Autodesk Fusion 360 part; units mm, degrees
note: some values were not read from the file. Set by a fixed rule: which sketch regions a step uses.
(part 12 of 14)
  spline S66 degree 5 poles (-8.0092, 17.6297) (-8.0092, 17.6297) (-8.0093, 17.6299) (-8.0094, 17.6301) (-8.0095, 17.6305) (-8.0098, 17.631) (-8.0101, 17.6317) (-8.0104, 17.6324) (-8.0108, 17.6332) (-8.0112, 17.634) (-8.0117, 17.635) (-8.0122, 17.636) (-8.0127, 17.6371) (-8.0133, 17.6383) (-8.0139, 17.6395) (-8.0146, 17.6408) (-8.0153, 17.6422) (-8.016, 17.6437) (-8.0168, 17.6452) (-8.0176, 17.6469) (-8.0185, 17.6485) (-8.0194, 17.6503) (-8.0203, 17.6521) (-8.0213, 17.654) (-8.0223, 17.6559) (-8.0234, 17.6579) (-8.0245, 17.66) (-8.0256, 17.6621) (-8.0268, 17.6643) (-8.028, 17.6666) (-8.0292, 17.6689) (-8.0305, 17.6713) (-8.0318, 17.6737) (-8.0332, 17.6762) (-8.0346, 17.6788) (-8.0361, 17.6814) (-8.0375, 17.6841) (-8.0391, 17.6868) (-8.0406, 17.6896) (-8.0422, 17.6925) (-8.0438, 17.6954) (-8.0455, 17.6983) (-8.0472, 17.7013) (-8.049, 17.7044) (-8.0508, 17.7075) (-8.0526, 17.7107) (-8.0545, 17.7139) (-8.0564, 17.7172) (-8.0583, 17.7205) (-8.0603, 17.7239) (-8.0623, 17.7273) (-8.0644, 17.7308) (-8.0665, 17.7343) (-8.0686, 17.7378) (-8.0708, 17.7415) (-8.073, 17.7451) (-8.0752, 17.7488) (-8.0775, 17.7526) (-8.0798, 17.7564) (-8.0822, 17.7602) (-8.0846, 17.7641) (-8.087, 17.7681) (-8.0895, 17.772) (-8.092, 17.7761) (-8.0945, 17.7801) (-8.0971, 17.7842) (-8.0997, 17.7884) (-8.1024, 17.7926) (-8.1051, 17.7968) (-8.1078, 17.8011) (-8.1106, 17.8054) (-8.1134, 17.8097) (-8.1162, 17.8141) (-8.1191, 17.8186) (-8.122, 17.823) (-8.125, 17.8276) (-8.128, 17.8321) (-8.131, 17.8367) (-8.1341, 17.8413) (-8.1372, 17.846) (-8.1403, 17.8507) (-8.1435, 17.8554) (-8.1467, 17.8602) (-8.1499, 17.865) (-8.1532, 17.8698) (-8.1565, 17.8747) (-8.1599, 17.8796) (-8.1633, 17.8846) (-8.1667, 17.8896) (-8.1702, 17.8946) (-8.1737, 17.8996) (-8.1772, 17.9047) (-8.1808, 17.9098) (-8.1844, 17.915) (-8.1881, 17.9202) (-8.1918, 17.9254) (-8.1955, 17.9306) (-8.1993, 17.9359) (-8.2031, 17.9412) (-8.2069, 17.9466) (-8.2108, 17.9519) (-8.2147, 17.9573) (-8.2186, 17.9628) (-8.2226, 17.9682) (-8.2266, 17.9737) (-8.2306, 17.9793) (-8.2347, 17.9848) (-8.2388, 17.9904) (-8.243, 17.996) (-8.2472, 18.0016) (-8.2514, 18.0073) (-8.2557, 18.013) (-8.26, 18.0187) (-8.2643, 18.0244) (-8.2687, 18.0302) (-8.2731, 18.036) (-8.2775, 18.0418) (-8.282, 18.0477) (-8.2865, 18.0536) (-8.291, 18.0595) (-8.2956, 18.0654) (-8.3003, 18.0714) (-8.3049, 18.0773) (-8.3096, 18.0833) (-8.3143, 18.0894) (-8.3191, 18.0954) (-8.3239, 18.1015) (-8.3287, 18.1076) (-8.3336, 18.1137) (-8.3385, 18.1199) (-8.3434, 18.126) (-8.3484, 18.1322) (-8.3534, 18.1385) (-8.3584, 18.1447) (-8.3635, 18.151) (-8.3686, 18.1572) (-8.3737, 18.1635) (-8.3789, 18.1699) (-8.3841, 18.1762) (-8.3894, 18.1826) (-8.3947, 18.189) (-8.4, 18.1954) (-8.4054, 18.2018) (-8.4107, 18.2083) (-8.4162, 18.2148) (-8.4216, 18.2213) (-8.4271, 18.2278) (-8.4326, 18.2343) (-8.4382, 18.2409) (-8.4438, 18.2474) (-8.4494, 18.254) (-8.4551, 18.2606) (-8.4608, 18.2673) (-8.4665, 18.2739) (-8.4723, 18.2806) (-8.4781, 18.2873) (-8.4839, 18.294) (-8.4898, 18.3007) (-8.4957, 18.3074) (-8.5017, 18.3142) (-8.5076, 18.321) (-8.5137, 18.3277) (-8.5197, 18.3346) (-8.5258, 18.3414) (-8.5319, 18.3482) (-8.538, 18.3551) (-8.5442, 18.3619) (-8.5504, 18.3688) (-8.5567, 18.3757) (-8.5629, 18.3827) (-8.5693, 18.3896) (-8.5756, 18.3966) (-8.582, 18.4035) (-8.5884, 18.4105) (-8.5949, 18.4175) (-8.6013, 18.4245) (-8.6079, 18.4315) (-8.6144, 18.4386) (-8.621, 18.4456) (-8.6276, 18.4527) (-8.6343, 18.4598) (-8.641, 18.4669) (-8.6477, 18.474) (-8.6544, 18.4811) (-8.6612, 18.4883) (-8.668, 18.4954) (-8.6749, 18.5026) (-8.6818, 18.5098) (-8.6887, 18.517) (-8.6956, 18.5242) (-8.7026, 18.5314) (-8.7096, 18.5386) (-8.7167, 18.5459) (-8.7238, 18.5531) (-8.7309, 18.5604) (-8.7381, 18.5677) (-8.7452, 18.575) (-8.7525, 18.5823) (-8.7597, 18.5896) (-8.767, 18.5969) (-8.7743, 18.6042) (-8.7817, 18.6116) (-8.789, 18.6189) (-8.7965, 18.6263) (-8.8039, 18.6337) (-8.8114, 18.6411) (-8.8189, 18.6485) (-8.8264, 18.6559) (-8.834, 18.6633) (-8.8416, 18.6707) (-8.8493, 18.6782) (-8.857, 18.6856) (-8.8647, 18.6931) (-8.8724, 18.7005) (-8.8802, 18.708) (-8.888, 18.7155) (-8.8958, 18.723) (-8.9037, 18.7305) (-8.9116, 18.738) (-8.9195, 18.7455) (-8.9275, 18.7531) (-8.9355, 18.7606) (-8.9436, 18.7681) (-8.9516, 18.7757) (-8.9597, 18.7833) (-8.9678, 18.7908) (-8.976, 18.7984) (-8.9842, 18.806) (-8.9924, 18.8136) (-9.0007, 18.8212) (-9.009, 18.8288) (-9.0173, 18.8364) (-9.0257, 18.844) (-9.034, 18.8517) (-9.0425, 18.8593) (-9.0509, 18.8669) (-9.0594, 18.8746) (-9.0679, 18.8823) (-9.0765, 18.8899) (-9.085, 18.8976) (-9.0936, 18.9053) (-9.1006, 18.9114) (-9.1058, 18.916) (-9.1092, 18.9191) (-9.111, 18.9206) knots 0 0 0 0 0 0 0.00416667 0.00833333 0.0125 0.01666667 0.02083333 0.025 0.02916667 0.03333333 0.0375 0.04166667 0.04583333 0.05 0.05416667 0.05833333 0.0625 0.06666667 0.07083333 0.075 0.07916667 0.08333333 0.0875 0.09166667 0.09583333 0.1 0.10416667 0.10833333 0.1125 0.11666667 0.12083333 0.125 0.12916667 0.13333333 0.1375 0.14166667 0.14583333 0.15 0.15416667 0.15833333 0.1625 0.16666667 0.17083333 0.175 0.17916667 0.18333333 0.1875 0.19166667 0.19583333 0.2 0.20416667 0.20833333 0.2125 0.21666667 0.22083333 0.225 0.22916667 0.23333333 0.2375 0.24166667 0.24583333 0.25 0.25416667 0.25833333 0.2625 0.26666667 0.27083333 0.275 0.27916667 0.28333333 0.2875 0.29166667 0.29583333 0.3 0.30416667 0.30833333 0.3125 0.31666667 0.32083333 0.325 0.32916667 0.33333333 0.3375 0.34166667 0.34583333 0.35 0.35416667 0.35833333 0.3625 0.36666667 0.37083333 0.375 0.37916667 0.38333333 0.3875 0.39166667 0.39583333 0.4 0.40416667 0.40833333 0.4125 0.41666667 0.42083333 0.425 0.42916667 0.43333333 0.4375 0.44166667 0.44583333 0.45 0.45416667 0.45833333 0.4625 0.46666667 0.47083333 0.475 0.47916667 0.48333333 0.4875 0.49166667 0.49583333 0.5 0.50416667 0.50833333 0.5125 0.51666667 0.52083333 0.525 0.52916667 0.53333333 0.5375 0.54166667 0.54583333 0.55 0.55416667 0.55833333 0.5625 0.56666667 0.57083333 0.575 0.57916667 0.58333333 0.5875 0.59166667 0.59583333 0.6 0.60416667 0.60833333 0.6125 0.61666667 0.62083333 0.625 0.62916667 0.63333333 0.6375 0.64166667 0.64583333 0.65 0.65416667 0.65833333 0.6625 0.66666667 0.67083333 0.675 0.67916667 0.68333333 0.6875 0.69166667 0.69583333 0.7 0.70416667 0.70833333 0.7125 0.71666667 0.72083333 0.725 0.72916667 0.73333333 0.7375 0.74166667 0.74583333 0.75 0.75416667 0.75833333 0.7625 0.76666667 0.77083333 0.775 0.77916667 0.78333333 0.7875 0.79166667 0.79583333 0.8 0.80416667 0.80833333 0.8125 0.81666667 0.82083333 0.825 0.82916667 0.83333333 0.8375 0.84166667 0.84583333 0.85 0.85416667 0.85833333 0.8625 0.86666667 0.87083333 0.875 0.87916667 0.88333333 0.8875 0.89166667 0.89583333 0.9 0.90416667 0.90833333 0.9125 0.91666667 0.92083333 0.925 0.92916667 0.93333333 0.9375 0.94166667 0.94583333 0.95 0.95416667 0.95833333 0.9625 0.96666667 0.97083333 0.975 0.97916667 0.98333333 0.9875 0.99166667 0.99583333 1 1 1 1 1 1
  arc A67 (-9.111, 18.9206) -> (-9.9518, 18.4922) centre (0, 0) ccw
  spline S67 degree 5 poles (-9.9518, 18.4922) (-9.9516, 18.4899) (-9.9512, 18.4853) (-9.9505, 18.4783) (-9.9496, 18.4691) (-9.9484, 18.4577) (-9.9473, 18.4462) (-9.9461, 18.4348) (-9.9449, 18.4234) (-9.9437, 18.4121) (-9.9425, 18.4007) (-9.9412, 18.3894) (-9.94, 18.3782) (-9.9387, 18.3669) (-9.9375, 18.3557) (-9.9362, 18.3445) (-9.9349, 18.3334) (-9.9336, 18.3223) (-9.9323, 18.3112) (-9.9309, 18.3001) (-9.9296, 18.2891) (-9.9282, 18.2781) (-9.9269, 18.2671) (-9.9255, 18.2562) (-9.9241, 18.2453) (-9.9227, 18.2344) (-9.9213, 18.2236) (-9.9198, 18.2128) (-9.9184, 18.202) (-9.9169, 18.1912) (-9.9155, 18.1805) (-9.914, 18.1698) (-9.9125, 18.1592) (-9.911, 18.1486) (-9.9095, 18.138) (-9.9079, 18.1274) (-9.9064, 18.1169) (-9.9049, 18.1064) (-9.9033, 18.0959) (-9.9017, 18.0855) (-9.9002, 18.0751) (-9.8986, 18.0647) (-9.897, 18.0544) (-9.8953, 18.0441) (-9.8937, 18.0339) (-9.8921, 18.0236) (-9.8904, 18.0134) (-9.8888, 18.0033) (-9.8871, 17.9931) (-9.8855, 17.983) (-9.8838, 17.973) (-9.8821, 17.9629) (-9.8804, 17.9529) (-9.8787, 17.943) (-9.8769, 17.9331) (-9.8752, 17.9232) (-9.8735, 17.9133) (-9.8717, 17.9035) (-9.8699, 17.8937) (-9.8682, 17.8839) (-9.8664, 17.8742) (-9.8646, 17.8645) (-9.8628, 17.8549) (-9.861, 17.8453) (-9.8592, 17.8357) (-9.8574, 17.8261) (-9.8555, 17.8166) (-9.8537, 17.8071) (-9.8519, 17.7977) (-9.85, 17.7883) (-9.8481, 17.7789) (-9.8463, 17.7696) (-9.8444, 17.7603) (-9.8425, 17.751) (-9.8406, 17.7418) (-9.8387, 17.7326) (-9.8368, 17.7235) (-9.8349, 17.7144) (-9.833, 17.7053) (-9.831, 17.6963) (-9.8291, 17.6873) (-9.8272, 17.6783) (-9.8252, 17.6694) (-9.8233, 17.6605) (-9.8213, 17.6516) (-9.8193, 17.6428) (-9.8174, 17.634) (-9.8154, 17.6253) (-9.8134, 17.6166) (-9.8114, 17.6079) (-9.8094, 17.5993) (-9.8074, 17.5907) (-9.8054, 17.5822) (-9.8034, 17.5737) (-9.8014, 17.5652) (-9.7993, 17.5568) (-9.7973, 17.5484) (-9.7953, 17.54) (-9.7932, 17.5317) (-9.7912, 17.5234) (-9.7892, 17.5152) (-9.7871, 17.507) (-9.785, 17.4988) (-9.783, 17.4907) (-9.7809, 17.4827) (-9.7789, 17.4746) (-9.7768, 17.4666) (-9.7747, 17.4587) (-9.7727, 17.4508) (-9.7706, 17.4429) (-9.7685, 17.4351) (-9.7664, 17.4273) (-9.7643, 17.4195) (-9.7622, 17.4118) (-9.7602, 17.4042) (-9.7581, 17.3966) (-9.756, 17.389) (-9.7539, 17.3814) (-9.7518, 17.3739) (-9.7497, 17.3665) (-9.7476, 17.3591) (-9.7455, 17.3517) (-9.7434, 17.3444) (-9.7413, 17.3371) (-9.7392, 17.3299) (-9.7371, 17.3227) (-9.735, 17.3155) (-9.7329, 17.3084) (-9.7308, 17.3014) (-9.7287, 17.2944) (-9.7265, 17.2874) (-9.7244, 17.2805) (-9.7223, 17.2736) (-9.7202, 17.2667) (-9.7181, 17.2599) (-9.7161, 17.2532) (-9.714, 17.2465) (-9.7119, 17.2398) (-9.7098, 17.2332) (-9.7077, 17.2267) (-9.7056, 17.2201) (-9.7035, 17.2137) (-9.7014, 17.2072) (-9.6993, 17.2009) (-9.6973, 17.1945) (-9.6952, 17.1882) (-9.6931, 17.182) (-9.6911, 17.1758) (-9.689, 17.1697) (-9.6869, 17.1636) (-9.6849, 17.1575) (-9.6828, 17.1515) (-9.6808, 17.1456) (-9.6788, 17.1397) (-9.6767, 17.1338) (-9.6747, 17.128) (-9.6727, 17.1223) (-9.6707, 17.1166) (-9.6687, 17.1109) (-9.6667, 17.1053) (-9.6647, 17.0997) (-9.6627, 17.0942) (-9.6607, 17.0888) (-9.6587, 17.0834) (-9.6568, 17.078) (-9.6548, 17.0727) (-9.6528, 17.0675) (-9.6509, 17.0623) (-9.649, 17.0571) (-9.6471, 17.052) (-9.6451, 17.047) (-9.6432, 17.042) (-9.6413, 17.0371) (-9.6395, 17.0322) (-9.6376, 17.0273) (-9.6357, 17.0226) (-9.6339, 17.0178) (-9.632, 17.0132) (-9.6302, 17.0086) (-9.6284, 17.004) (-9.6266, 16.9995) (-9.6248, 16.9951) (-9.623, 16.9907) (-9.6212, 16.9863) (-9.6195, 16.982) (-9.6177, 16.9778) (-9.616, 16.9737) (-9.6143, 16.9695) (-9.6126, 16.9655) (-9.6109, 16.9615) (-9.6093, 16.9576) (-9.6076, 16.9537) (-9.606, 16.9499) (-9.6044, 16.9461) (-9.6028, 16.9424) (-9.6012, 16.9387) (-9.5996, 16.9352) (-9.5981, 16.9316) (-9.5966, 16.9282) (-9.5951, 16.9248) (-9.5936, 16.9214) (-9.5921, 16.9182) (-9.5906, 16.9149) (-9.5892, 16.9118) (-9.5878, 16.9087) (-9.5864, 16.9057) (-9.5851, 16.9027) (-9.5837, 16.8998) (-9.5824, 16.897) (-9.5811, 16.8942) (-9.5798, 16.8915) (-9.5786, 16.8888) (-9.5774, 16.8863) (-9.5762, 16.8837) (-9.575, 16.8813) (-9.5739, 16.8789) (-9.5727, 16.8766) (-9.5716, 16.8744) (-9.5706, 16.8722) (-9.5695, 16.8701) (-9.5685, 16.8681) (-9.5676, 16.8661) (-9.5666, 16.8642) (-9.5657, 16.8624) (-9.5648, 16.8606) (-9.564, 16.859) (-9.5631, 16.8574) (-9.5624, 16.8558) (-9.5616, 16.8544) (-9.5609, 16.853) (-9.5602, 16.8517) (-9.5596, 16.8504) (-9.5589, 16.8493) (-9.5584, 16.8482) (-9.5578, 16.8472) (-9.5573, 16.8462) (-9.5569, 16.8454) (-9.5565, 16.8446) (-9.5561, 16.8439) (-9.5558, 16.8433) (-9.5555, 16.8428) (-9.5553, 16.8424) (-9.5551, 16.8422) (-9.5551, 16.8421) (-9.555, 16.842) knots -1 -1 -1 -1 -1 -1 -0.99583333 -0.99166667 -0.9875 -0.98333333 -0.97916667 -0.975 -0.97083333 -0.96666667 -0.9625 -0.95833333 -0.95416667 -0.95 -0.94583333 -0.94166667 -0.9375 -0.93333333 -0.92916667 -0.925 -0.92083333 -0.91666667 -0.9125 -0.90833333 -0.90416667 -0.9 -0.89583333 -0.89166667 -0.8875 -0.88333333 -0.87916667 -0.875 -0.87083333 -0.86666667 -0.8625 -0.85833333 -0.85416667 -0.85 -0.84583333 -0.84166667 -0.8375 -0.83333333 -0.82916667 -0.825 -0.82083333 -0.81666667 -0.8125 -0.80833333 -0.80416667 -0.8 -0.79583333 -0.79166667 -0.7875 -0.78333333 -0.77916667 -0.775 -0.77083333 -0.76666667 -0.7625 -0.75833333 -0.75416667 -0.75 -0.74583333 -0.74166667 -0.7375 -0.73333333 -0.72916667 -0.725 -0.72083333 -0.71666667 -0.7125 -0.70833333 -0.70416667 -0.7 -0.69583333 -0.69166667 -0.6875 -0.68333333 -0.67916667 -0.675 -0.67083333 -0.66666667 -0.6625 -0.65833333 -0.65416667 -0.65 -0.64583333 -0.64166667 -0.6375 -0.63333333 -0.62916667 -0.625 -0.62083333 -0.61666667 -0.6125 -0.60833333 -0.60416667 -0.6 -0.59583333 -0.59166667 -0.5875 -0.58333333 -0.57916667 -0.575 -0.57083333 -0.56666667 -0.5625 -0.55833333 -0.55416667 -0.55 -0.54583333 -0.54166667 -0.5375 -0.53333333 -0.52916667 -0.525 -0.52083333 -0.51666667 -0.5125 -0.50833333 -0.50416667 -0.5 -0.49583333 -0.49166667 -0.4875 -0.48333333 -0.47916667 -0.475 -0.47083333 -0.46666667 -0.4625 -0.45833333 -0.45416667 -0.45 -0.44583333 -0.44166667 -0.4375 -0.43333333 -0.42916667 -0.425 -0.42083333 -0.41666667 -0.4125 -0.40833333 -0.40416667 -0.4 -0.39583333 -0.39166667 -0.3875 -0.38333333 -0.37916667 -0.375 -0.37083333 -0.36666667 -0.3625 -0.35833333 -0.35416667 -0.35 -0.34583333 -0.34166667 -0.3375 -0.33333333 -0.32916667 -0.325 -0.32083333 -0.31666667 -0.3125 -0.30833333 -0.30416667 -0.3 -0.29583333 -0.29166667 -0.2875 -0.28333333 -0.27916667 -0.275 -0.27083333 -0.26666667 -0.2625 -0.25833333 -0.25416667 -0.25 -0.24583333 -0.24166667 -0.2375 -0.23333333 -0.22916667 -0.225 -0.22083333 -0.21666667 -0.2125 -0.20833333 -0.20416667 -0.2 -0.19583333 -0.19166667 -0.1875 -0.18333333 -0.17916667 -0.175 -0.17083333 -0.16666667 -0.1625 -0.15833333 -0.15416667 -0.15 -0.14583333 -0.14166667 -0.1375 -0.13333333 -0.12916667 -0.125 -0.12083333 -0.11666667 -0.1125 -0.10833333 -0.10416667 -0.1 -0.09583333 -0.09166667 -0.0875 -0.08333333 -0.07916667 -0.075 -0.07083333 -0.06666667 -0.0625 -0.05833333 -0.05416667 -0.05 -0.04583333 -0.04166667 -0.0375 -0.03333333 -0.02916667 -0.025 -0.02083333 -0.01666667 -0.0125 -0.00833333 -0.00416667 0 0 0 0 0 0
  line L134 (-9.555, 16.842) -> (-9.5547, 16.8414)
  line L135 (-9.5547, 16.8414) -> (-9.2522, 16.3082)
  arc A68 (-9.2522, 16.3082) -> (-10.3303, 15.6476) centre (0, 0) ccw
  line L136 (-10.3303, 15.6476) -> (-10.668, 16.1591)
  line L137 (-10.668, 16.1591) -> (-10.6684, 16.1597)
  spline S68 degree 5 poles (-10.6684, 16.1597) (-10.6685, 16.1598) (-10.6686, 16.1599) (-10.6687, 16.1601) (-10.6689, 16.1605) (-10.6693, 16.1609) (-10.6697, 16.1615) (-10.6701, 16.1622) (-10.6706, 16.1629) (-10.6712, 16.1637) (-10.6718, 16.1646) (-10.6724, 16.1655) (-10.6731, 16.1665) (-10.6739, 16.1676) (-10.6747, 16.1687) (-10.6756, 16.1699) (-10.6765, 16.1712) (-10.6774, 16.1725) (-10.6784, 16.1739) (-10.6795, 16.1754) (-10.6806, 16.1769) (-10.6818, 16.1785) (-10.683, 16.1801) (-10.6842, 16.1818) (-10.6855, 16.1836) (-10.6869, 16.1854) (-10.6883, 16.1873) (-10.6897, 16.1892) (-10.6912, 16.1912) (-10.6928, 16.1932) (-10.6944, 16.1953) (-10.696, 16.1975) (-10.6977, 16.1997) (-10.6995, 16.202) (-10.7013, 16.2043) (-10.7031, 16.2066) (-10.705, 16.209) (-10.7069, 16.2115) (-10.7089, 16.214) (-10.7109, 16.2166) (-10.713, 16.2192) (-10.7151, 16.2218) (-10.7173, 16.2245) (-10.7195, 16.2273) (-10.7217, 16.2301) (-10.724, 16.2329) (-10.7264, 16.2358) (-10.7288, 16.2388) (-10.7312, 16.2417) (-10.7337, 16.2448) (-10.7362, 16.2478) (-10.7388, 16.2509) (-10.7414, 16.2541) (-10.7441, 16.2573) (-10.7468, 16.2605) (-10.7495, 16.2638) (-10.7523, 16.2671) (-10.7552, 16.2704) (-10.7581, 16.2738) (-10.761, 16.2772) (-10.764, 16.2807) (-10.767, 16.2842) (-10.77, 16.2878) (-10.7731, 16.2913) (-10.7763, 16.295) (-10.7795, 16.2986) (-10.7827, 16.3023) (-10.786, 16.306) (-10.7893, 16.3098) (-10.7927, 16.3136) (-10.7961, 16.3174) (-10.7996, 16.3213) (-10.8031, 16.3252) (-10.8066, 16.3291) (-10.8102, 16.333) (-10.8138, 16.337) (-10.8175, 16.3411) (-10.8212, 16.3451) (-10.8249, 16.3492) (-10.8287, 16.3533) (-10.8325, 16.3575) (-10.8364, 16.3617) (-10.8403, 16.3659) (-10.8443, 16.3701) (-10.8483, 16.3744) (-10.8524, 16.3787) (-10.8564, 16.383) (-10.8606, 16.3874) (-10.8647, 16.3918) (-10.8689, 16.3962) (-10.8732, 16.4006) (-10.8775, 16.4051) (-10.8818, 16.4096) (-10.8862, 16.4141) (-10.8906, 16.4187) (-10.8951, 16.4232) (-10.8996, 16.4278) (-10.9041, 16.4325) (-10.9087, 16.4371) (-10.9133, 16.4418) (-10.918, 16.4465) (-10.9227, 16.4512) (-10.9274, 16.456) (-10.9322, 16.4607) (-10.937, 16.4655) (-10.9419, 16.4703) (-10.9468, 16.4752) (-10.9517, 16.4801) (-10.9567, 16.4849) (-10.9617, 16.4899) (-10.9668, 16.4948) (-10.9719, 16.4997) (-10.977, 16.5047) (-10.9822, 16.5097) (-10.9874, 16.5147) (-10.9927, 16.5198) (-10.998, 16.5248) (-11.0033, 16.5299) (-11.0087, 16.535) (-11.0141, 16.5401) (-11.0196, 16.5453) (-11.025, 16.5504) (-11.0306, 16.5556) (-11.0361, 16.5608) (-11.0418, 16.566) (-11.0474, 16.5712) (-11.0531, 16.5765) (-11.0588, 16.5818) (-11.0646, 16.5871) (-11.0704, 16.5924) (-11.0762, 16.5977) (-11.0821, 16.603) (-11.088, 16.6084) (-11.094, 16.6138) (-11.1, 16.6192) (-11.106, 16.6246) (-11.1121, 16.63) (-11.1182, 16.6354) (-11.1243, 16.6409) (-11.1305, 16.6463) (-11.1367, 16.6518) (-11.143, 16.6573) (-11.1493, 16.6629) (-11.1556, 16.6684) (-11.162, 16.6739) (-11.1684, 16.6795) (-11.1748, 16.6851) (-11.1813, 16.6907) (-11.1878, 16.6963) (-11.1944, 16.7019) (-11.201, 16.7075) (-11.2076, 16.7131) (-11.2143, 16.7188) (-11.221, 16.7245) (-11.2277, 16.7302) (-11.2345, 16.7358) (-11.2413, 16.7416) (-11.2482, 16.7473) (-11.255, 16.753) (-11.262, 16.7587) (-11.2689, 16.7645) (-11.2759, 16.7703) (-11.283, 16.7761) (-11.29, 16.7818) (-11.2971, 16.7876) (-11.3043, 16.7935) (-11.3115, 16.7993) (-11.3187, 16.8051) (-11.3259, 16.811) (-11.3332, 16.8168) (-11.3405, 16.8227) (-11.3479, 16.8285) (-11.3553, 16.8344) (-11.3627, 16.8403) (-11.3702, 16.8462) (-11.3777, 16.8521) (-11.3852, 16.8581) (-11.3928, 16.864) (-11.4004, 16.8699) (-11.408, 16.8759) (-11.4157, 16.8818) (-11.4234, 16.8878) (-11.4312, 16.8938) (-11.439, 16.8998) (-11.4468, 16.9057) (-11.4546, 16.9117) (-11.4625, 16.9178) (-11.4705, 16.9238) (-11.4784, 16.9298) (-11.4864, 16.9358) (-11.4944, 16.9419) (-11.5025, 16.9479) (-11.5106, 16.9539) (-11.5187, 16.96) (-11.5269, 16.9661) (-11.5351, 16.9721) (-11.5433, 16.9782) (-11.5516, 16.9843) (-11.5599, 16.9904) (-11.5683, 16.9965) (-11.5766, 17.0026) (-11.585, 17.0087) (-11.5935, 17.0148) (-11.602, 17.0209) (-11.6105, 17.027) (-11.619, 17.0332) (-11.6276, 17.0393) (-11.6362, 17.0454) (-11.6448, 17.0516) (-11.6535, 17.0577) (-11.6622, 17.0639) (-11.671, 17.07) (-11.6798, 17.0762) (-11.6886, 17.0823) (-11.6974, 17.0885) (-11.7063, 17.0947) (-11.7152, 17.1009) (-11.7242, 17.107) (-11.7332, 17.1132) (-11.7422, 17.1194) (-11.7512, 17.1256) (-11.7603, 17.1318) (-11.7694, 17.138) (-11.7786, 17.1442) (-11.7878, 17.1504) (-11.797, 17.1566) (-11.8062, 17.1628) (-11.8155, 17.169) (-11.8248, 17.1752) (-11.8342, 17.1815) (-11.8435, 17.1877) (-11.8529, 17.1939) (-11.8624, 17.2001) (-11.8719, 17.2063) (-11.8814, 17.2126) (-11.8909, 17.2188) (-11.9005, 17.225) (-11.9101, 17.2312) (-11.9197, 17.2375) (-11.9294, 17.2437) (-11.9391, 17.2499) (-11.9469, 17.2549) (-11.9528, 17.2587) (-11.9567, 17.2612) (-11.9586, 17.2624) knots 0 0 0 0 0 0 0.00416667 0.00833333 0.0125 0.01666667 0.02083333 0.025 0.02916667 0.03333333 0.0375 0.04166667 0.04583333 0.05 0.05416667 0.05833333 0.0625 0.06666667 0.07083333 0.075 0.07916667 0.08333333 0.0875 0.09166667 0.09583333 0.1 0.10416667 0.10833333 0.1125 0.11666667 0.12083333 0.125 0.12916667 0.13333333 0.1375 0.14166667 0.14583333 0.15 0.15416667 0.15833333 0.1625 0.16666667 0.17083333 0.175 0.17916667 0.18333333 0.1875 0.19166667 0.19583333 0.2 0.20416667 0.20833333 0.2125 0.21666667 0.22083333 0.225 0.22916667 0.23333333 0.2375 0.24166667 0.24583333 0.25 0.25416667 0.25833333 0.2625 0.26666667 0.27083333 0.275 0.27916667 0.28333333 0.2875 0.29166667 0.29583333 0.3 0.30416667 0.30833333 0.3125 0.31666667 0.32083333 0.325 0.32916667 0.33333333 0.3375 0.34166667 0.34583333 0.35 0.35416667 0.35833333 0.3625 0.36666667 0.37083333 0.375 0.37916667 0.38333333 0.3875 0.39166667 0.39583333 0.4 0.40416667 0.40833333 0.4125 0.41666667 0.42083333 0.425 0.42916667 0.43333333 0.4375 0.44166667 0.44583333 0.45 0.45416667 0.45833333 0.4625 0.46666667 0.47083333 0.475 0.47916667 0.48333333 0.4875 0.49166667 0.49583333 0.5 0.50416667 0.50833333 0.5125 0.51666667 0.52083333 0.525 0.52916667 0.53333333 0.5375 0.54166667 0.54583333 0.55 0.55416667 0.55833333 0.5625 0.56666667 0.57083333 0.575 0.57916667 0.58333333 0.5875 0.59166667 0.59583333 0.6 0.60416667 0.60833333 0.6125 0.61666667 0.62083333 0.625 0.62916667 0.63333333 0.6375 0.64166667 0.64583333 0.65 0.65416667 0.65833333 0.6625 0.66666667 0.67083333 0.675 0.67916667 0.68333333 0.6875 0.69166667 0.69583333 0.7 0.70416667 0.70833333 0.7125 0.71666667 0.72083333 0.725 0.72916667 0.73333333 0.7375 0.74166667 0.74583333 0.75 0.75416667 0.75833333 0.7625 0.76666667 0.77083333 0.775 0.77916667 0.78333333 0.7875 0.79166667 0.79583333 0.8 0.80416667 0.80833333 0.8125 0.81666667 0.82083333 0.825 0.82916667 0.83333333 0.8375 0.84166667 0.84583333 0.85 0.85416667 0.85833333 0.8625 0.86666667 0.87083333 0.875 0.87916667 0.88333333 0.8875 0.89166667 0.89583333 0.9 0.90416667 0.90833333 0.9125 0.91666667 0.92083333 0.925 0.92916667 0.93333333 0.9375 0.94166667 0.94583333 0.95 0.95416667 0.95833333 0.9625 0.96666667 0.97083333 0.975 0.97916667 0.98333333 0.9875 0.99166667 0.99583333 1 1 1 1 1 1
  arc A69 (-11.9586, 17.2624) -> (-12.7221, 16.7077) centre (0, 0) ccw
  spline S69 degree 5 poles (-12.7221, 16.7077) (-12.7215, 16.7055) (-12.7204, 16.701) (-12.7186, 16.6943) (-12.7163, 16.6853) (-12.7134, 16.6741) (-12.7104, 16.663) (-12.7075, 16.6519) (-12.7045, 16.6409) (-12.7015, 16.6298) (-12.6986, 16.6188) (-12.6956, 16.6079) (-12.6926, 16.5969) (-12.6896, 16.586) (-12.6866, 16.5752) (-12.6836, 16.5643) (-12.6806, 16.5535) (-12.6775, 16.5427) (-12.6745, 16.532) (-12.6714, 16.5213) (-12.6684, 16.5106) (-12.6653, 16.4999) (-12.6622, 16.4893) (-12.6592, 16.4787) (-12.6561, 16.4682) (-12.653, 16.4577) (-12.6499, 16.4472) (-12.6468, 16.4367) (-12.6437, 16.4263) (-12.6406, 16.4159) (-12.6374, 16.4056) (-12.6343, 16.3952) (-12.6312, 16.385) (-12.628, 16.3747) (-12.6249, 16.3645) (-12.6217, 16.3543) (-12.6185, 16.3441) (-12.6154, 16.334) (-12.6122, 16.3239) (-12.609, 16.3139) (-12.6058, 16.3038) (-12.6026, 16.2939) (-12.5994, 16.2839) (-12.5962, 16.274) (-12.593, 16.2641) (-12.5898, 16.2543) (-12.5866, 16.2444) (-12.5834, 16.2347) (-12.5801, 16.2249) (-12.5769, 16.2152) (-12.5737, 16.2055) (-12.5704, 16.1959) (-12.5672, 16.1863) (-12.5639, 16.1767) (-12.5607, 16.1672) (-12.5574, 16.1577) (-12.5542, 16.1482) (-12.5509, 16.1388) (-12.5476, 16.1294) (-12.5443, 16.12) (-12.5411, 16.1107) (-12.5378, 16.1014) (-12.5345, 16.0922) (-12.5312, 16.0829) (-12.5279, 16.0738) (-12.5246, 16.0646) (-12.5213, 16.0555) (-12.518, 16.0464) (-12.5147, 16.0374) (-12.5114, 16.0284) (-12.5081, 16.0195) (-12.5048, 16.0105) (-12.5015, 16.0016) (-12.4982, 15.9928) (-12.4949, 15.984) (-12.4916, 15.9752) (-12.4883, 15.9665) (-12.4849, 15.9578) (-12.4816, 15.9491) (-12.4783, 15.9405) (-12.475, 15.9319) (-12.4717, 15.9233) (-12.4683, 15.9148) (-12.465, 15.9063) (-12.4617, 15.8979) (-12.4584, 15.8895) (-12.4551, 15.8811) (-12.4517, 15.8728) (-12.4484, 15.8645) (-12.4451, 15.8563) (-12.4418, 15.8481) (-12.4384, 15.8399) (-12.4351, 15.8318) (-12.4318, 15.8237) (-12.4285, 15.8157) (-12.4252, 15.8076) (-12.4219, 15.7997) (-12.4185, 15.7917) (-12.4152, 15.7839) (-12.4119, 15.776) (-12.4086, 15.7682) (-12.4053, 15.7604) (-12.402, 15.7527) (-12.3987, 15.745) (-12.3954, 15.7373) (-12.3921, 15.7297) (-12.3888, 15.7222) (-12.3855, 15.7146) (-12.3822, 15.7071) (-12.379, 15.6997) (-12.3757, 15.6923) (-12.3724, 15.6849) (-12.3691, 15.6776) (-12.3659, 15.6703) (-12.3626, 15.6631) (-12.3593, 15.6559) (-12.3561, 15.6487) (-12.3528, 15.6416) (-12.3496, 15.6345) (-12.3464, 15.6275) (-12.3431, 15.6205) (-12.3399, 15.6136) (-12.3367, 15.6067) (-12.3335, 15.5998) (-12.3303, 15.593) (-12.3271, 15.5862) (-12.3239, 15.5795) (-12.3207, 15.5728) (-12.3175, 15.5661) (-12.3143, 15.5595) (-12.3111, 15.553) (-12.308, 15.5465) (-12.3048, 15.54) (-12.3017, 15.5336) (-12.2986, 15.5272) (-12.2954, 15.5209) (-12.2923, 15.5146) (-12.2892, 15.5083) (-12.2861, 15.5021) (-12.283, 15.496) (-12.2799, 15.4898) (-12.2769, 15.4838) (-12.2738, 15.4778) (-12.2707, 15.4718) (-12.2677, 15.4658) (-12.2647, 15.46) (-12.2616, 15.4541) (-12.2586, 15.4483) (-12.2556, 15.4426) (-12.2527, 15.4369) (-12.2497, 15.4312) (-12.2467, 15.4256) (-12.2438, 15.4201) (-12.2408, 15.4146) (-12.2379, 15.4091) (-12.235, 15.4037) (-12.2321, 15.3983) (-12.2292, 15.393) (-12.2264, 15.3877) (-12.2235, 15.3825) (-12.2207, 15.3773) (-12.2178, 15.3722) (-12.215, 15.3671) (-12.2122, 15.3621) (-12.2095, 15.3571) (-12.2067, 15.3522) (-12.2039, 15.3473) (-12.2012, 15.3425) (-12.1985, 15.3377) (-12.1958, 15.333) (-12.1931, 15.3283) (-12.1905, 15.3236) (-12.1878, 15.3191) (-12.1852, 15.3145) (-12.1826, 15.3101) (-12.18, 15.3056) (-12.1774, 15.3013) (-12.1749, 15.2969) (-12.1724, 15.2927) (-12.1699, 15.2884) (-12.1674, 15.2843) (-12.1649, 15.2802) (-12.1625, 15.2761) (-12.16, 15.2721) (-12.1576, 15.2681) (-12.1553, 15.2642) (-12.1529, 15.2604) (-12.1506, 15.2566) (-12.1483, 15.2529) (-12.146, 15.2492) (-12.1437, 15.2456) (-12.1415, 15.242) (-12.1393, 15.2385) (-12.1371, 15.235) (-12.1349, 15.2316) (-12.1328, 15.2282) (-12.1307, 15.2249) (-12.1286, 15.2217) (-12.1266, 15.2185) (-12.1245, 15.2154) (-12.1225, 15.2123) (-12.1206, 15.2093) (-12.1186, 15.2064) (-12.1167, 15.2035) (-12.1149, 15.2007) (-12.113, 15.1979) (-12.1112, 15.1952) (-12.1094, 15.1925) (-12.1077, 15.1899) (-12.106, 15.1874) (-12.1043, 15.1849) (-12.1027, 15.1825) (-12.101, 15.1801) (-12.0995, 15.1778) (-12.0979, 15.1756) (-12.0964, 15.1734) (-12.095, 15.1713) (-12.0935, 15.1693) (-12.0921, 15.1673) (-12.0908, 15.1654) (-12.0895, 15.1635) (-12.0882, 15.1618) (-12.087, 15.16) (-12.0858, 15.1584) (-12.0846, 15.1568) (-12.0835, 15.1553) (-12.0825, 15.1538) (-12.0815, 15.1524) (-12.0805, 15.1511) (-12.0796, 15.1498) (-12.0787, 15.1486) (-12.0778, 15.1475) (-12.0771, 15.1465) (-12.0763, 15.1455) (-12.0756, 15.1446) (-12.075, 15.1437) (-12.0744, 15.143) (-12.0739, 15.1423) (-12.0734, 15.1417) (-12.073, 15.1411) (-12.0726, 15.1406) (-12.0724, 15.1403) (-12.0722, 15.1401) (-12.0721, 15.14) (-12.0721, 15.1399) knots -1 -1 -1 -1 -1 -1 -0.99583333 -0.99166667 -0.9875 -0.98333333 -0.97916667 -0.975 -0.97083333 -0.96666667 -0.9625 -0.95833333 -0.95416667 -0.95 -0.94583333 -0.94166667 -0.9375 -0.93333333 -0.92916667 -0.925 -0.92083333 -0.91666667 -0.9125 -0.90833333 -0.90416667 -0.9 -0.89583333 -0.89166667 -0.8875 -0.88333333 -0.87916667 -0.875 -0.87083333 -0.86666667 -0.8625 -0.85833333 -0.85416667 -0.85 -0.84583333 -0.84166667 -0.8375 -0.83333333 -0.82916667 -0.825 -0.82083333 -0.81666667 -0.8125 -0.80833333 -0.80416667 -0.8 -0.79583333 -0.79166667 -0.7875 -0.78333333 -0.77916667 -0.775 -0.77083333 -0.76666667 -0.7625 -0.75833333 -0.75416667 -0.75 -0.74583333 -0.74166667 -0.7375 -0.73333333 -0.72916667 -0.725 -0.72083333 -0.71666667 -0.7125 -0.70833333 -0.70416667 -0.7 -0.69583333 -0.69166667 -0.6875 -0.68333333 -0.67916667 -0.675 -0.67083333 -0.66666667 -0.6625 -0.65833333 -0.65416667 -0.65 -0.64583333 -0.64166667 -0.6375 -0.63333333 -0.62916667 -0.625 -0.62083333 -0.61666667 -0.6125 -0.60833333 -0.60416667 -0.6 -0.59583333 -0.59166667 -0.5875 -0.58333333 -0.57916667 -0.575 -0.57083333 -0.56666667 -0.5625 -0.55833333 -0.55416667 -0.55 -0.54583333 -0.54166667 -0.5375 -0.53333333 -0.52916667 -0.525 -0.52083333 -0.51666667 -0.5125 -0.50833333 -0.50416667 -0.5 -0.49583333 -0.49166667 -0.4875 -0.48333333 -0.47916667 -0.475 -0.47083333 -0.46666667 -0.4625 -0.45833333 -0.45416667 -0.45 -0.44583333 -0.44166667 -0.4375 -0.43333333 -0.42916667 -0.425 -0.42083333 -0.41666667 -0.4125 -0.40833333 -0.40416667 -0.4 -0.39583333 -0.39166667 -0.3875 -0.38333333 -0.37916667 -0.375 -0.37083333 -0.36666667 -0.3625 -0.35833333 -0.35416667 -0.35 -0.34583333 -0.34166667 -0.3375 -0.33333333 -0.32916667 -0.325 -0.32083333 -0.31666667 -0.3125 -0.30833333 -0.30416667 -0.3 -0.29583333 -0.29166667 -0.2875 -0.28333333 -0.27916667 -0.275 -0.27083333 -0.26666667 -0.2625 -0.25833333 -0.25416667 -0.25 -0.24583333 -0.24166667 -0.2375 -0.23333333 -0.22916667 -0.225 -0.22083333 -0.21666667 -0.2125 -0.20833333 -0.20416667 -0.2 -0.19583333 -0.19166667 -0.1875 -0.18333333 -0.17916667 -0.175 -0.17083333 -0.16666667 -0.1625 -0.15833333 -0.15416667 -0.15 -0.14583333 -0.14166667 -0.1375 -0.13333333 -0.12916667 -0.125 -0.12083333 -0.11666667 -0.1125 -0.10833333 -0.10416667 -0.1 -0.09583333 -0.09166667 -0.0875 -0.08333333 -0.07916667 -0.075 -0.07083333 -0.06666667 -0.0625 -0.05833333 -0.05416667 -0.05 -0.04583333 -0.04166667 -0.0375 -0.03333333 -0.02916667 -0.025 -0.02083333 -0.01666667 -0.0125 -0.00833333 -0.00416667 0 0 0 0 0 0
  line L138 (-12.0721, 15.1399) -> (-12.0716, 15.1394)
  line L139 (-12.0716, 15.1394) -> (-11.6895, 14.6601)
  arc A70 (-11.6895, 14.6601) -> (-12.651, 13.8389) centre (0, 0) ccw
  line L140 (-12.651, 13.8389) -> (-13.0645, 14.2913)
  line L141 (-13.0645, 14.2913) -> (-13.065, 14.2918)
  spline S70 degree 5 poles (-13.065, 14.2918) (-13.0651, 14.2919) (-13.0652, 14.292) (-13.0654, 14.2922) (-13.0656, 14.2925) (-13.0661, 14.2929) (-13.0665, 14.2934) (-13.0671, 14.294) (-13.0677, 14.2946) (-13.0684, 14.2953) (-13.0691, 14.2961) (-13.0699, 14.2969) (-13.0707, 14.2978) (-13.0716, 14.2987) (-13.0726, 14.2997) (-13.0737, 14.3008) (-13.0747, 14.3019) (-13.0759, 14.3031) (-13.0771, 14.3043) (-13.0784, 14.3056) (-13.0797, 14.3069) (-13.0811, 14.3083) (-13.0826, 14.3097) (-13.0841, 14.3112) (-13.0856, 14.3127) (-13.0873, 14.3143) (-13.089, 14.316) (-13.0907, 14.3176) (-13.0925, 14.3194) (-13.0943, 14.3212) (-13.0962, 14.323) (-13.0982, 14.3248) (-13.1002, 14.3268) (-13.1023, 14.3287) (-13.1044, 14.3307) (-13.1066, 14.3328) (-13.1088, 14.3349) (-13.1111, 14.337) (-13.1135, 14.3392) (-13.1159, 14.3414) (-13.1183, 14.3436) (-13.1208, 14.3459) (-13.1234, 14.3482) (-13.126, 14.3506) (-13.1287, 14.353) (-13.1314, 14.3555) (-13.1342, 14.358) (-13.137, 14.3605) (-13.1398, 14.363) (-13.1428, 14.3656) (-13.1457, 14.3683) (-13.1488, 14.3709) (-13.1519, 14.3736) (-13.155, 14.3764) (-13.1582, 14.3791) (-13.1614, 14.3819) (-13.1647, 14.3848) (-13.168, 14.3876) (-13.1714, 14.3905) (-13.1748, 14.3935) (-13.1783, 14.3964) (-13.1818, 14.3994) (-13.1854, 14.4024) (-13.189, 14.4055) (-13.1927, 14.4086) (-13.1964, 14.4117) (-13.2002, 14.4148) (-13.204, 14.418) (-13.2079, 14.4212) (-13.2118, 14.4244) (-13.2158, 14.4276) (-13.2198, 14.4309) (-13.2239, 14.4342) (-13.228, 14.4375) (-13.2321, 14.4409) (-13.2363, 14.4443) (-13.2406, 14.4477) (-13.2449, 14.4511) (-13.2492, 14.4545) (-13.2536, 14.458) (-13.2581, 14.4615) (-13.2625, 14.465) (-13.2671, 14.4686) (-13.2716, 14.4722) (-13.2763, 14.4758) (-13.2809, 14.4794) (-13.2856, 14.483) (-13.2904, 14.4867) (-13.2952, 14.4903) (-13.3001, 14.494) (-13.305, 14.4978) (-13.3099, 14.5015) (-13.3149, 14.5053) (-13.3199, 14.509) (-13.325, 14.5128) (-13.3301, 14.5167) (-13.3353, 14.5205) (-13.3405, 14.5244) (-13.3457, 14.5282) (-13.351, 14.5321) (-13.3563, 14.5361) (-13.3617, 14.54) (-13.3672, 14.5439) (-13.3726, 14.5479) (-13.3781, 14.5519) (-13.3837, 14.5559) (-13.3893, 14.5599) (-13.3949, 14.5639) (-13.4006, 14.568) (-13.4063, 14.572) (-13.4121, 14.5761) (-13.4179, 14.5802) (-13.4238, 14.5843) (-13.4297, 14.5885) (-13.4356, 14.5926) (-13.4416, 14.5967) (-13.4476, 14.6009) (-13.4537, 14.6051) (-13.4598, 14.6093) (-13.4659, 14.6135) (-13.4721, 14.6177) (-13.4784, 14.622) (-13.4846, 14.6262) (-13.491, 14.6305) (-13.4973, 14.6347) (-13.5037, 14.639) (-13.5101, 14.6433) (-13.5166, 14.6476) (-13.5231, 14.652) (-13.5297, 14.6563) (-13.5363, 14.6606) (-13.5429, 14.665) (-13.5496, 14.6694) (-13.5563, 14.6737) (-13.5631, 14.6781) (-13.5699, 14.6825) (-13.5768, 14.6869) (-13.5836, 14.6913) (-13.5906, 14.6958) (-13.5975, 14.7002) (-13.6045, 14.7047) (-13.6116, 14.7091) (-13.6186, 14.7136) (-13.6258, 14.718) (-13.6329, 14.7225) (-13.6401, 14.727) (-13.6474, 14.7315) (-13.6546, 14.736) (-13.6619, 14.7405) (-13.6693, 14.7451) (-13.6767, 14.7496) (-13.6841, 14.7541) (-13.6916, 14.7587) (-13.6991, 14.7632) (-13.7067, 14.7678) (-13.7142, 14.7723) (-13.7219, 14.7769) (-13.7295, 14.7815) (-13.7372, 14.7861) (-13.745, 14.7907) (-13.7527, 14.7953) (-13.7605, 14.7999) (-13.7684, 14.8045) (-13.7763, 14.8091) (-13.7842, 14.8137) (-13.7922, 14.8183) (-13.8002, 14.8229) (-13.8082, 14.8276) (-13.8163, 14.8322) (-13.8244, 14.8369) (-13.8326, 14.8415) (-13.8407, 14.8462) (-13.849, 14.8508) (-13.8572, 14.8555) (-13.8655, 14.8601) (-13.8739, 14.8648) (-13.8822, 14.8695) (-13.8906, 14.8741) (-13.8991, 14.8788) (-13.9076, 14.8835) (-13.9161, 14.8882) (-13.9246, 14.8929) (-13.9332, 14.8976) (-13.9418, 14.9022) (-13.9505, 14.9069) (-13.9592, 14.9116) (-13.9679, 14.9163) (-13.9767, 14.921) (-13.9855, 14.9257) (-13.9943, 14.9304) (-14.0032, 14.9351) (-14.0121, 14.9398) (-14.0211, 14.9446) (-14.03, 14.9493) (-14.0391, 14.954) (-14.0481, 14.9587) (-14.0572, 14.9634) (-14.0663, 14.9681) (-14.0755, 14.9728) (-14.0847, 14.9775) (-14.0939, 14.9823) (-14.1031, 14.987) (-14.1124, 14.9917) (-14.1218, 14.9964) (-14.1311, 15.0011) (-14.1405, 15.0058) (-14.15, 15.0105) (-14.1594, 15.0153) (-14.1689, 15.02) (-14.1785, 15.0247) (-14.188, 15.0294) (-14.1976, 15.0341) (-14.2073, 15.0388) (-14.2169, 15.0435) (-14.2267, 15.0482) (-14.2364, 15.053) (-14.2462, 15.0577) (-14.256, 15.0624) (-14.2658, 15.0671) (-14.2757, 15.0718) (-14.2856, 15.0765) (-14.2955, 15.0812) (-14.3055, 15.0859) (-14.3155, 15.0905) (-14.3255, 15.0952) (-14.3356, 15.0999) (-14.3457, 15.1046) (-14.3559, 15.1093) (-14.366, 15.114) (-14.3762, 15.1186) (-14.3865, 15.1233) (-14.3967, 15.128) (-14.407, 15.1327) (-14.4174, 15.1373) (-14.4277, 15.142) (-14.4381, 15.1466) (-14.4486, 15.1513) (-14.459, 15.156) (-14.4695, 15.1606) (-14.4801, 15.1652) (-14.4906, 15.1699) (-14.4991, 15.1736) (-14.5055, 15.1764) (-14.5097, 15.1782) (-14.5118, 15.1792) knots 0 0 0 0 0 0 0.00416667 0.00833333 0.0125 0.01666667 0.02083333 0.025 0.02916667 0.03333333 0.0375 0.04166667 0.04583333 0.05 0.05416667 0.05833333 0.0625 0.06666667 0.07083333 0.075 0.07916667 0.08333333 0.0875 0.09166667 0.09583333 0.1 0.10416667 0.10833333 0.1125 0.11666667 0.12083333 0.125 0.12916667 0.13333333 0.1375 0.14166667 0.14583333 0.15 0.15416667 0.15833333 0.1625 0.16666667 0.17083333 0.175 0.17916667 0.18333333 0.1875 0.19166667 0.19583333 0.2 0.20416667 0.20833333 0.2125 0.21666667 0.22083333 0.225 0.22916667 0.23333333 0.2375 0.24166667 0.24583333 0.25 0.25416667 0.25833333 0.2625 0.26666667 0.27083333 0.275 0.27916667 0.28333333 0.2875 0.29166667 0.29583333 0.3 0.30416667 0.30833333 0.3125 0.31666667 0.32083333 0.325 0.32916667 0.33333333 0.3375 0.34166667 0.34583333 0.35 0.35416667 0.35833333 0.3625 0.36666667 0.37083333 0.375 0.37916667 0.38333333 0.3875 0.39166667 0.39583333 0.4 0.40416667 0.40833333 0.4125 0.41666667 0.42083333 0.425 0.42916667 0.43333333 0.4375 0.44166667 0.44583333 0.45 0.45416667 0.45833333 0.4625 0.46666667 0.47083333 0.475 0.47916667 0.48333333 0.4875 0.49166667 0.49583333 0.5 0.50416667 0.50833333 0.5125 0.51666667 0.52083333 0.525 0.52916667 0.53333333 0.5375 0.54166667 0.54583333 0.55 0.55416667 0.55833333 0.5625 0.56666667 0.57083333 0.575 0.57916667 0.58333333 0.5875 0.59166667 0.59583333 0.6 0.60416667 0.60833333 0.6125 0.61666667 0.62083333 0.625 0.62916667 0.63333333 0.6375 0.64166667 0.64583333 0.65 0.65416667 0.65833333 0.6625 0.66666667 0.67083333 0.675 0.67916667 0.68333333 0.6875 0.69166667 0.69583333 0.7 0.70416667 0.70833333 0.7125 0.71666667 0.72083333 0.725 0.72916667 0.73333333 0.7375 0.74166667 0.74583333 0.75 0.75416667 0.75833333 0.7625 0.76666667 0.77083333 0.775 0.77916667 0.78333333 0.7875 0.79166667 0.79583333 0.8 0.80416667 0.80833333 0.8125 0.81666667 0.82083333 0.825 0.82916667 0.83333333 0.8375 0.84166667 0.84583333 0.85 0.85416667 0.85833333 0.8625 0.86666667 0.87083333 0.875 0.87916667 0.88333333 0.8875 0.89166667 0.89583333 0.9 0.90416667 0.90833333 0.9125 0.91666667 0.92083333 0.925 0.92916667 0.93333333 0.9375 0.94166667 0.94583333 0.95 0.95416667 0.95833333 0.9625 0.96666667 0.97083333 0.975 0.97916667 0.98333333 0.9875 0.99166667 0.99583333 1 1 1 1 1 1
  arc A71 (-14.5118, 15.1792) -> (-15.1792, 14.5118) centre (0, 0) ccw
  spline S71 degree 5 poles (-15.1792, 14.5118) (-15.1782, 14.5097) (-15.1764, 14.5055) (-15.1736, 14.4991) (-15.1699, 14.4906) (-15.1652, 14.4801) (-15.1606, 14.4695) (-15.156, 14.459) (-15.1513, 14.4486) (-15.1466, 14.4381) (-15.142, 14.4277) (-15.1373, 14.4174) (-15.1327, 14.407) (-15.128, 14.3967) (-15.1233, 14.3865) (-15.1186, 14.3762) (-15.114, 14.366) (-15.1093, 14.3559) (-15.1046, 14.3457) (-15.0999, 14.3356) (-15.0952, 14.3255) (-15.0905, 14.3155) (-15.0859, 14.3055) (-15.0812, 14.2955) (-15.0765, 14.2856) (-15.0718, 14.2757) (-15.0671, 14.2658) (-15.0624, 14.256) (-15.0577, 14.2462) (-15.053, 14.2364) (-15.0482, 14.2267) (-15.0435, 14.2169) (-15.0388, 14.2073) (-15.0341, 14.1976) (-15.0294, 14.188) (-15.0247, 14.1785) (-15.02, 14.1689) (-15.0153, 14.1594) (-15.0105, 14.15) (-15.0058, 14.1405) (-15.0011, 14.1311) (-14.9964, 14.1218) (-14.9917, 14.1124) (-14.987, 14.1031) (-14.9823, 14.0939) (-14.9775, 14.0847) (-14.9728, 14.0755) (-14.9681, 14.0663) (-14.9634, 14.0572) (-14.9587, 14.0481) (-14.954, 14.0391) (-14.9493, 14.03) (-14.9446, 14.0211) (-14.9398, 14.0121) (-14.9351, 14.0032) (-14.9304, 13.9943) (-14.9257, 13.9855) (-14.921, 13.9767) (-14.9163, 13.9679) (-14.9116, 13.9592) (-14.9069, 13.9505) (-14.9022, 13.9418) (-14.8976, 13.9332) (-14.8929, 13.9246) (-14.8882, 13.9161) (-14.8835, 13.9076) (-14.8788, 13.8991) (-14.8741, 13.8906) (-14.8695, 13.8822) (-14.8648, 13.8739) (-14.8601, 13.8655) (-14.8555, 13.8572) (-14.8508, 13.849) (-14.8462, 13.8407) (-14.8415, 13.8326) (-14.8369, 13.8244) (-14.8322, 13.8163) (-14.8276, 13.8082) (-14.8229, 13.8002) (-14.8183, 13.7922) (-14.8137, 13.7842) (-14.8091, 13.7763) (-14.8045, 13.7684) (-14.7999, 13.7605) (-14.7953, 13.7527) (-14.7907, 13.745) (-14.7861, 13.7372) (-14.7815, 13.7295) (-14.7769, 13.7219) (-14.7723, 13.7142) (-14.7678, 13.7067) (-14.7632, 13.6991) (-14.7587, 13.6916) (-14.7541, 13.6841) (-14.7496, 13.6767) (-14.7451, 13.6693) (-14.7405, 13.6619) (-14.736, 13.6546) (-14.7315, 13.6474) (-14.727, 13.6401) (-14.7225, 13.6329) (-14.718, 13.6258) (-14.7136, 13.6186) (-14.7091, 13.6116) (-14.7047, 13.6045) (-14.7002, 13.5975) (-14.6958, 13.5906) (-14.6913, 13.5836) (-14.6869, 13.5768) (-14.6825, 13.5699) (-14.6781, 13.5631) (-14.6737, 13.5563) (-14.6694, 13.5496) (-14.665, 13.5429) (-14.6606, 13.5363) (-14.6563, 13.5297) (-14.652, 13.5231) (-14.6476, 13.5166) (-14.6433, 13.5101) (-14.639, 13.5037) (-14.6347, 13.4973) (-14.6305, 13.491) (-14.6262, 13.4846) (-14.622, 13.4784) (-14.6177, 13.4721) (-14.6135, 13.4659) (-14.6093, 13.4598) (-14.6051, 13.4537) (-14.6009, 13.4476) (-14.5967, 13.4416) (-14.5926, 13.4356) (-14.5885, 13.4297) (-14.5843, 13.4238) (-14.5802, 13.4179) (-14.5761, 13.4121) (-14.572, 13.4063) (-14.568, 13.4006) (-14.5639, 13.3949) (-14.5599, 13.3893) (-14.5559, 13.3837) (-14.5519, 13.3781) (-14.5479, 13.3726) (-14.5439, 13.3672) (-14.54, 13.3617) (-14.5361, 13.3563) (-14.5321, 13.351) (-14.5282, 13.3457) (-14.5244, 13.3405) (-14.5205, 13.3353) (-14.5167, 13.3301) (-14.5128, 13.325) (-14.509, 13.3199) (-14.5053, 13.3149) (-14.5015, 13.3099) (-14.4978, 13.305) (-14.494, 13.3001) (-14.4903, 13.2952) (-14.4867, 13.2904) (-14.483, 13.2856) (-14.4794, 13.2809) (-14.4758, 13.2763) (-14.4722, 13.2716) (-14.4686, 13.2671) (-14.465, 13.2625) (-14.4615, 13.2581) (-14.458, 13.2536) (-14.4545, 13.2492) (-14.4511, 13.2449) (-14.4477, 13.2406) (-14.4443, 13.2363) (-14.4409, 13.2321) (-14.4375, 13.228) (-14.4342, 13.2239) (-14.4309, 13.2198) (-14.4276, 13.2158) (-14.4244, 13.2118) (-14.4212, 13.2079) (-14.418, 13.204) (-14.4148, 13.2002) (-14.4117, 13.1964) (-14.4086, 13.1927) (-14.4055, 13.189) (-14.4024, 13.1854) (-14.3994, 13.1818) (-14.3964, 13.1783) (-14.3935, 13.1748) (-14.3905, 13.1714) (-14.3876, 13.168) (-14.3848, 13.1647) (-14.3819, 13.1614) (-14.3791, 13.1582) (-14.3764, 13.155) (-14.3736, 13.1519) (-14.3709, 13.1488) (-14.3683, 13.1457) (-14.3656, 13.1428) (-14.363, 13.1398) (-14.3605, 13.137) (-14.358, 13.1342) (-14.3555, 13.1314) (-14.353, 13.1287) (-14.3506, 13.126) (-14.3482, 13.1234) (-14.3459, 13.1208) (-14.3436, 13.1183) (-14.3414, 13.1159) (-14.3392, 13.1135) (-14.337, 13.1111) (-14.3349, 13.1088) (-14.3328, 13.1066) (-14.3307, 13.1044) (-14.3287, 13.1023) (-14.3268, 13.1002) (-14.3248, 13.0982) (-14.323, 13.0962) (-14.3212, 13.0943) (-14.3194, 13.0925) (-14.3176, 13.0907) (-14.316, 13.089) (-14.3143, 13.0873) (-14.3127, 13.0856) (-14.3112, 13.0841) (-14.3097, 13.0826) (-14.3083, 13.0811) (-14.3069, 13.0797) (-14.3056, 13.0784) (-14.3043, 13.0771) (-14.3031, 13.0759) (-14.3019, 13.0747) (-14.3008, 13.0737) (-14.2997, 13.0726) (-14.2987, 13.0716) (-14.2978, 13.0707) (-14.2969, 13.0699) (-14.2961, 13.0691) (-14.2953, 13.0684) (-14.2946, 13.0677) (-14.294, 13.0671) (-14.2934, 13.0665) (-14.2929, 13.0661) (-14.2925, 13.0656) (-14.2922, 13.0654) (-14.292, 13.0652) (-14.2919, 13.0651) (-14.2918, 13.065) knots -1 -1 -1 -1 -1 -1 -0.99583333 -0.99166667 -0.9875 -0.98333333 -0.97916667 -0.975 -0.97083333 -0.96666667 -0.9625 -0.95833333 -0.95416667 -0.95 -0.94583333 -0.94166667 -0.9375 -0.93333333 -0.92916667 -0.925 -0.92083333 -0.91666667 -0.9125 -0.90833333 -0.90416667 -0.9 -0.89583333 -0.89166667 -0.8875 -0.88333333 -0.87916667 -0.875 -0.87083333 -0.86666667 -0.8625 -0.85833333 -0.85416667 -0.85 -0.84583333 -0.84166667 -0.8375 -0.83333333 -0.82916667 -0.825 -0.82083333 -0.81666667 -0.8125 -0.80833333 -0.80416667 -0.8 -0.79583333 -0.79166667 -0.7875 -0.78333333 -0.77916667 -0.775 -0.77083333 -0.76666667 -0.7625 -0.75833333 -0.75416667 -0.75 -0.74583333 -0.74166667 -0.7375 -0.73333333 -0.72916667 -0.725 -0.72083333 -0.71666667 -0.7125 -0.70833333 -0.70416667 -0.7 -0.69583333 -0.69166667 -0.6875 -0.68333333 -0.67916667 -0.675 -0.67083333 -0.66666667 -0.6625 -0.65833333 -0.65416667 -0.65 -0.64583333 -0.64166667 -0.6375 -0.63333333 -0.62916667 -0.625 -0.62083333 -0.61666667 -0.6125 -0.60833333 -0.60416667 -0.6 -0.59583333 -0.59166667 -0.5875 -0.58333333 -0.57916667 -0.575 -0.57083333 -0.56666667 -0.5625 -0.55833333 -0.55416667 -0.55 -0.54583333 -0.54166667 -0.5375 -0.53333333 -0.52916667 -0.525 -0.52083333 -0.51666667 -0.5125 -0.50833333 -0.50416667 -0.5 -0.49583333 -0.49166667 -0.4875 -0.48333333 -0.47916667 -0.475 -0.47083333 -0.46666667 -0.4625 -0.45833333 -0.45416667 -0.45 -0.44583333 -0.44166667 -0.4375 -0.43333333 -0.42916667 -0.425 -0.42083333 -0.41666667 -0.4125 -0.40833333 -0.40416667 -0.4 -0.39583333 -0.39166667 -0.3875 -0.38333333 -0.37916667 -0.375 -0.37083333 -0.36666667 -0.3625 -0.35833333 -0.35416667 -0.35 -0.34583333 -0.34166667 -0.3375 -0.33333333 -0.32916667 -0.325 -0.32083333 -0.31666667 -0.3125 -0.30833333 -0.30416667 -0.3 -0.29583333 -0.29166667 -0.2875 -0.28333333 -0.27916667 -0.275 -0.27083333 -0.26666667 -0.2625 -0.25833333 -0.25416667 -0.25 -0.24583333 -0.24166667 -0.2375 -0.23333333 -0.22916667 -0.225 -0.22083333 -0.21666667 -0.2125 -0.20833333 -0.20416667 -0.2 -0.19583333 -0.19166667 -0.1875 -0.18333333 -0.17916667 -0.175 -0.17083333 -0.16666667 -0.1625 -0.15833333 -0.15416667 -0.15 -0.14583333 -0.14166667 -0.1375 -0.13333333 -0.12916667 -0.125 -0.12083333 -0.11666667 -0.1125 -0.10833333 -0.10416667 -0.1 -0.09583333 -0.09166667 -0.0875 -0.08333333 -0.07916667 -0.075 -0.07083333 -0.06666667 -0.0625 -0.05833333 -0.05416667 -0.05 -0.04583333 -0.04166667 -0.0375 -0.03333333 -0.02916667 -0.025 -0.02083333 -0.01666667 -0.0125 -0.00833333 -0.00416667 0 0 0 0 0 0
  line L142 (-14.2918, 13.065) -> (-14.2913, 13.0645)
  line L143 (-14.2913, 13.0645) -> (-13.8389, 12.651)
  arc A72 (-13.8389, 12.651) -> (-14.6601, 11.6895) centre (0, 0) ccw
  line L144 (-14.6601, 11.6895) -> (-15.1394, 12.0716)
  line L145 (-15.1394, 12.0716) -> (-15.1399, 12.0721)